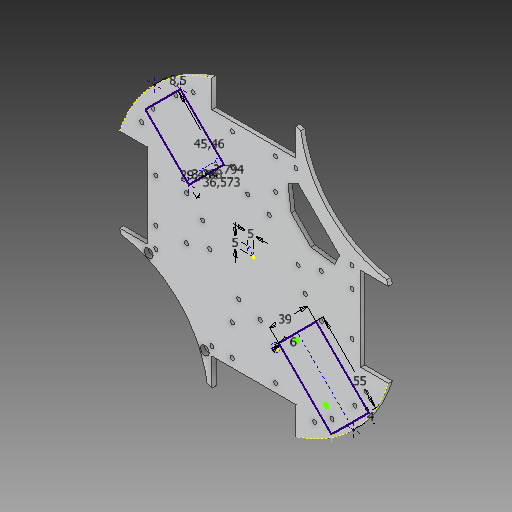
# Autodesk Inventor part: floor-01
Saved by Autodesk Inventor 2020 (Build 240168000, 168)
## iProperties
Created: 2024-09-07
Part Number: floor-01
Material: Типовые
Document SubType Name: Modeling
Designer: Ivan
Density: 1 g/cm^3
Appearance: С текстурой — серый
Author: Ivan
Autodesk Inventor part; units mm, degrees
ref_plane "YZ Plane" through (0, 0, 0) normal (1, 0, 0) x (0, 1, 0)
ref_plane "XZ Plane" through (0, 0, 0) normal (0, 1, 0) x (-1, 0, 0)
ref_plane "XY Plane" through (0, 0, 0) normal (0, 0, 1) x (1, 0, 0)
sketch "Эскиз2" plane through (0, 0, 0) normal (0, 0, 1) x (1, 0, 0)
  circle A0 centre (0, 0) radius 107.5
  circle A1 centre (0, 0) radius 104
  line L0 (-99.2724, 31) -> (-78.7724, 31)
  line L1 (-99.2724, -31) -> (-78.7724, -31)
  line L2 (-31, 99.2724) -> (-31, 78.7724)
  line L3 (31, 99.2724) -> (31, 78.7724)
  line L4 (99.2724, 31) -> (78.7724, 31)
  line L5 (99.2724, -31) -> (78.7724, -31)
  line L6 (31, -99.2724) -> (31, -78.7724)
  line L7 (-31, -99.2724) -> (-31, -78.7724)
  line L8 (-78.7724, -31) -> (-78.7724, 31)
  line L9 (-31, 78.7724) -> (31, 78.7724)
  line L10 (78.7724, 31) -> (78.7724, -31)
  line L11 (31, -78.7724) -> (-31, -78.7724)
  circle A2 centre (-109.0212, -109.0212) radius 75.25
  line L12 (-31, 78.7724) -> (78.7724, -31) construction
  line L13 (-73.5391, 73.5391) -> (73.5391, -73.5391) construction
  circle A3 centre (109.0212, 109.0212) radius 75.25
  point P0 (-98.0863, -34.57)
  point P1 (-34.57, -98.0863)
  point P2 (98.0863, 34.57)
  point P3 (34.57, 98.0863)
  dimension "d1" = 208
  dimension "d0" = 215
  dimension "d8" = 20.5
  dimension "d9" = 31
  dimension "d10" = 31
  dimension "d11" = 31
  dimension "d12" = 31
  dimension "d13" = 31
  dimension "d14" = 31
  dimension "d15" = 31
  dimension "d16" = 31
  dimension "d17" = 150.5
  dimension "d18" = 3.57
  dimension "d19" = 3.57
  constraints: 28 end point, 7 equal length, 4 horizontal, 4 vertical, 3 centre point, 2 coincident, 2 point on circle, 1 midpoint, 1 parallel, 1 symmetric about line, 15 other
  measures "d0" diameter of A0
  measures "d8" distance of L0.start L0.end
  measures "d9" distance from line of L0 point (0, 0)
  measures "d10" distance from line of L7 point (0, 0)
  measures "d11" distance from line of L6 point (0, 0)
  measures "d12" distance from line of L5 point (0, 0)
  measures "d13" distance from line of L4 point (0, 0)
  measures "d14" distance from line of L3 point (0, 0)
  measures "d15" distance from line of L2 A0.centre
  measures "d16" distance from line of L1 point (0, 0)
  measures "d17" diameter of A2
  measures "d18" vertical distance of L1.start A2.end
  measures "d19" horizontal distance of L7.start A2.start
extrude "Выдавливание1" add sketch "Эскиз2" along normal blind 3 contours A1 L4 L10 L5 L6 L11 L7 A2 L1 L8 L0 L2 L9 L3 A3
sketch "Эскиз3" plane through (0, 0, 0) normal (0, 0, -1) x (-1, 0, 0)
  line L0 (-78.7724, -31) -> (-78.7724, 31) projected
  line L1 (-78.7724, 16) -> (78.7724, 16) construction
  line L2 (78.7724, 31) -> (78.7724, -31) projected
  line L3 (-31, 78.7724) -> (31, 78.7724) projected
  line L4 (31, -78.7724) -> (-31, -78.7724) projected
  line L5 (-16, -78.7724) -> (-16, 78.7724) construction
  line L6 (0, 0) -> (0, 78.7724) construction
  line L7 (0, 0) -> (78.7724, 0) construction
  line L8 (-78.7724, -16) -> (78.7724, -16) construction
  line L9 (16, -78.7724) -> (16, 78.7724) construction
  circle A0 centre (-49.72, 16) radius 1.5
  circle A1 centre (-49.72, -16) radius 1.5
  circle A2 centre (-16, 49.72) radius 1.5
  circle A3 centre (16, 49.72) radius 1.5
  circle A4 centre (49.72, 16) radius 1.5
  circle A5 centre (49.72, -16) radius 1.5
  line L10 (-49.72, 49.72) -> (49.72, 49.72) construction
  line L11 (49.72, 49.72) -> (49.72, -49.72) construction
  line L12 (49.72, -49.72) -> (-49.72, -49.72) construction
  line L13 (-49.72, -49.72) -> (-49.72, 49.72) construction
  line L14 (-49.72, 49.72) -> (49.72, -49.72) construction
  circle A6 centre (-16, -49.72) radius 1.5
  circle A7 centre (16, -49.72) radius 1.5
  line L15 (-72.43, 72.43) -> (72.43, 72.43) construction
  line L16 (72.43, 72.43) -> (72.43, -72.43) construction
  line L17 (72.43, -72.43) -> (-72.43, -72.43) construction
  line L18 (-72.43, -72.43) -> (-72.43, 72.43) construction
  line L19 (-72.43, 72.43) -> (72.43, -72.43) construction
  circle A8 centre (-72.43, 16) radius 1.5
  circle A9 centre (-72.43, -16) radius 1.5
  circle A10 centre (-16, 72.43) radius 1.5
  circle A11 centre (16, 72.43) radius 1.5
  circle A12 centre (72.43, 16) radius 1.5
  circle A13 centre (72.43, -16) radius 1.5
  circle A14 centre (16, -72.43) radius 1.5
  circle A15 centre (-16, -72.43) radius 1.5
  circle A16 centre (-72.43, 31) radius 1.5
  circle A17 centre (-31, 72.43) radius 1.5
  circle A18 centre (31, -72.43) radius 1.5
  circle A19 centre (72.43, -31) radius 1.5
  line L20 (-99.2724, -31) -> (-78.7724, -31) projected
  line L21 (-31, -78.7724) -> (-31, -99.2724) projected
  arc A20 (-89.0224, -31) -> (-31, -89.0224) centre (0, 0) ccw construction
  arc A21 (89.0224, 31) -> (31, 89.0224) centre (0, 0) ccw construction
  circle A22 centre (-57.67, -74.5664) radius 1.5
  line L22 (-72.43, -72.43) -> (72.43, 72.43) construction
  circle A23 centre (-74.5664, -57.67) radius 1.5
  circle A24 centre (-44.87, -82.9015) radius 1.5
  circle A25 centre (-82.9015, -44.87) radius 1.5
  circle A26 centre (74.5664, 57.67) radius 1.5
  circle A27 centre (57.67, 74.5664) radius 1.5
  circle A28 centre (82.9015, 44.87) radius 1.5
  circle A29 centre (44.87, 82.9015) radius 1.5
  dimension "d22" = 16
  dimension "d23" = 16
  dimension "d25" = 99.44
  dimension "d26" = 3
  dimension "d27" = 144.86
  dimension "d28" = 3
  dimension "d29" = 3
  dimension "d30" = 15
  dimension "d31" = 15
  dimension "d32" = 15
  dimension "d33" = 15
  dimension "d35" = 26.67
  dimension "d36" = 13.87
  dimension "d37" = 3
  constraints: 39 point on line, 34 end point, 30 centre point, 18 equal radius, 12 symmetric about line, 6 midpoint, 6 point on circle, 4 parallel, 4 perpendicular, 3 horizontal, 1 coincident, 1 vertical, 7 other
  measures "d22" distance from line of L1 L6.start
  measures "d23" distance from line of L5 L6.start
  measures "d25" distance of L11.end L12.end
  measures "d26" diameter of A0
  measures "d27" distance of L17.end L15.start
  measures "d28" diameter of A11
  measures "d29" diameter of A16
  measures "d30" distance of A16.centre A8.centre
  measures "d31" distance of A17.centre A10.centre
  measures "d32" distance of A13.centre A19.centre
  measures "d33" distance of A14.centre A18.centre
  measures "d35" distance from line of L21 A22.centre
  measures "d36" distance from line of L21 A24.centre
  measures "d37" diameter of A24
extrude "Выдавливание2" cut sketch "Эскиз3" against normal blind 3
sketch "Эскиз5" plane through (0, 0, 3) normal (0, 0, 1) x (1, 0, 0)
  circle A0 centre (16, -72.43) radius 1.5 projected
  circle A1 centre (16, -49.72) radius 1.5 projected
  circle A2 centre (49.72, -16) radius 1.5 projected
  circle A3 centre (49.72, 16) radius 1.5 projected
  circle A4 centre (72.43, 31) radius 1.5 projected
  circle A5 centre (-44.87, 82.9015) radius 1.5 projected
  circle A6 centre (57.67, -74.5664) radius 1.5 projected
  circle A7 centre (31, 72.43) radius 1.5 projected
  circle A8 centre (-57.67, 74.5664) radius 1.5 projected
  circle A9 centre (72.43, 16) radius 1.5 projected
  circle A10 centre (-49.72, 16) radius 1.5 projected
  circle A11 centre (-49.72, -16) radius 1.5 projected
  circle A12 centre (-16, -49.72) radius 1.5 projected
  circle A13 centre (74.5664, -57.67) radius 1.5 projected
  circle A14 centre (-16, -72.43) radius 1.5 projected
  circle A15 centre (-72.43, -31) radius 1.5 projected
  circle A16 centre (72.43, -16) radius 1.5 projected
  circle A17 centre (16, 49.72) radius 1.5 projected
  circle A18 centre (-82.9015, 44.87) radius 1.5 projected
  circle A19 centre (-16, 72.43) radius 1.5 projected
  circle A20 centre (44.87, -82.9015) radius 1.5 projected
  circle A21 centre (16, 72.43) radius 1.5 projected
  circle A22 centre (-74.5664, 57.67) radius 1.5 projected
  circle A23 centre (-16, 49.72) radius 1.5 projected
  circle A24 centre (-72.43, 16) radius 1.5 projected
  circle A25 centre (-72.43, -16) radius 1.5 projected
  circle A26 centre (-31, -72.43) radius 1.5 projected
  circle A27 centre (82.9015, -44.87) radius 1.5 projected
  arc A28 (-34.57, -98.0863) -> (-98.0863, -34.57) centre (-109.0212, -109.0212) ccw projected
  arc A29 (-34.57, -98.0863) -> (-31, -99.2724) centre (0, 0) ccw projected
  line L0 (-31, -99.2724) -> (-31, -78.7724) projected
  line L1 (-31, -78.7724) -> (31, -78.7724) projected
  line L2 (31, -78.7724) -> (31, -99.2724) projected
  arc A30 (31, -99.2724) -> (99.2724, -31) centre (0, 0) ccw projected
  line L3 (99.2724, -31) -> (78.7724, -31) projected
  line L4 (78.7724, -31) -> (78.7724, 31) projected
  line L5 (78.7724, 31) -> (99.2724, 31) projected
  arc A31 (99.2724, 31) -> (98.0863, 34.57) centre (0, 0) ccw projected
  arc A32 (34.57, 98.0863) -> (98.0863, 34.57) centre (109.0212, 109.0212) ccw projected
  arc A33 (34.57, 98.0863) -> (31, 99.2724) centre (0, 0) ccw projected
  line L6 (31, 99.2724) -> (31, 78.7724) projected
  line L7 (31, 78.7724) -> (-31, 78.7724) projected
  line L8 (-31, 78.7724) -> (-31, 99.2724) projected
  arc A34 (-31, 99.2724) -> (-99.2724, 31) centre (0, 0) ccw projected
  line L9 (-99.2724, 31) -> (-78.7724, 31) projected
  line L10 (-78.7724, 31) -> (-78.7724, -31) projected
  line L11 (-78.7724, -31) -> (-99.2724, -31) projected
  arc A35 (-99.2724, -31) -> (-98.0863, -34.57) centre (0, 0) ccw projected
  arc A36 (-31, 99.2724) -> (-99.2724, 31) centre (0, 0) ccw projected
  arc A37 (-31, 99.2724) -> (-99.2724, 31) centre (0, 0) ccw
  arc A38 (31, -99.2724) -> (99.2724, -31) centre (0, 0) ccw projected
  arc A39 (31, -99.2724) -> (99.2724, -31) centre (0, 0) ccw
  arc A40 (-34.57, -98.0863) -> (-98.0863, -34.57) centre (-109.0212, -109.0212) ccw projected
  arc A41 (-34.57, -98.0863) -> (-98.0863, -34.57) centre (-109.0212, -109.0212) ccw
  arc A42 (34.57, 98.0863) -> (98.0863, 34.57) centre (109.0212, 109.0212) ccw projected
  arc A43 (34.57, 98.0863) -> (98.0863, 34.57) centre (109.0212, 109.0212) ccw
  arc A44 (34.57, 98.0863) -> (31, 99.2724) centre (0, 0) ccw projected
  arc A45 (34.57, 98.0863) -> (31, 99.2724) centre (0, 0) ccw
  arc A46 (99.2724, 31) -> (98.0863, 34.57) centre (0, 0) ccw projected
  arc A47 (99.2724, 31) -> (98.0863, 34.57) centre (0, 0) ccw
  arc A48 (-34.57, -98.0863) -> (-31, -99.2724) centre (0, 0) ccw projected
  arc A49 (-34.57, -98.0863) -> (-31, -99.2724) centre (0, 0) ccw
  arc A50 (-99.2724, -31) -> (-98.0863, -34.57) centre (0, 0) ccw projected
  arc A51 (-99.2724, -31) -> (-98.0863, -34.57) centre (0, 0) ccw
  line L12 (-99.2724, 31) -> (-78.7724, 31) projected
  line L13 (-99.2724, 31) -> (-78.7724, 31)
  line L14 (-78.7724, 31) -> (-78.7724, -31) projected
  line L15 (-78.7724, 31) -> (-78.7724, -31)
  line L16 (-78.7724, -31) -> (-99.2724, -31)
  line L17 (-78.7724, -31) -> (-99.2724, -31) projected
  line L18 (-78.7724, -31) -> (-99.2724, -31)
  line L19 (-31, 78.7724) -> (-31, 99.2724) projected
  line L20 (-31, 99.2724) -> (-31, 78.7724)
  line L21 (31, 78.7724) -> (-31, 78.7724) projected
  line L22 (-31, 78.7724) -> (31, 78.7724)
  line L23 (31, 99.2724) -> (31, 78.7724) projected
  line L24 (31, 78.7724) -> (31, 99.2724)
  line L25 (78.7724, 31) -> (99.2724, 31) projected
  line L26 (99.2724, 31) -> (78.7724, 31)
  line L27 (78.7724, -31) -> (78.7724, 31) projected
  line L28 (78.7724, 31) -> (78.7724, -31)
  line L29 (99.2724, -31) -> (78.7724, -31) projected
  line L30 (78.7724, -31) -> (99.2724, -31)
  line L31 (-31, -99.2724) -> (-31, -78.7724) projected
  line L32 (-31, -99.2724) -> (-31, -78.7724)
  line L33 (-31, -78.7724) -> (31, -78.7724) projected
  line L34 (-31, -78.7724) -> (31, -78.7724)
  line L35 (31, -78.7724) -> (31, -99.2724)
  circle A52 centre (-49.72, 16) radius 1.5
  circle A53 centre (-72.43, 16) radius 1.5
  circle A54 centre (-49.72, -16) radius 1.5
  circle A55 centre (-72.43, -16) radius 1.5
  circle A56 centre (-72.43, -31) radius 1.5
  circle A57 centre (-16, -49.72) radius 1.5 projected
  circle A58 centre (-16, -49.72) radius 1.5
  circle A59 centre (-31, -72.43) radius 1.5 projected
  circle A60 centre (-31, -72.43) radius 1.5
  circle A61 centre (-16, -72.43) radius 1.5
  circle A62 centre (16, -72.43) radius 1.5 projected
  circle A63 centre (16, -72.43) radius 1.5
  circle A64 centre (44.87, -82.9015) radius 1.5
  circle A65 centre (57.67, -74.5664) radius 1.5
  circle A66 centre (16, -49.72) radius 1.5
  circle A67 centre (74.5664, -57.67) radius 1.5
  circle A68 centre (82.9015, -44.87) radius 1.5
  circle A69 centre (49.72, -16) radius 1.5
  circle A70 centre (72.43, -16) radius 1.5
  circle A71 centre (72.43, 16) radius 1.5
  circle A72 centre (49.72, 16) radius 1.5
  circle A73 centre (72.43, 31) radius 1.5
  circle A74 centre (31, 72.43) radius 1.5
  circle A75 centre (16, 72.43) radius 1.5
  circle A76 centre (16, 49.72) radius 1.5
  circle A77 centre (-16, 49.72) radius 1.5
  circle A78 centre (-16, 72.43) radius 1.5
  circle A79 centre (-44.87, 82.9015) radius 1.5
  circle A80 centre (-57.67, 74.5664) radius 1.5
  circle A81 centre (-74.5664, 57.67) radius 1.5
  circle A82 centre (-82.9015, 44.87) radius 1.5
  constraints: 36 centre point, 36 coincident, 26 end point, 19 concentric, 17 point on circle, 9 collinear, 1 horizontal, 1 perpendicular, 1 point on line
hole "Отверстие1" at (0, 0, 3) direction (0, 0, -1) diameter 40 end through all
sketch "Эскиз8" plane through (0, 0, 3) normal (0, 0, 1) x (1, 0, 0)
  circle A0 centre (-48.1257, 27.2915) radius 1.397 construction
  circle A1 centre (-27.2915, 48.1257) radius 1.397 construction
  line L0 (-48.3138, 22.4528) -> (-22.4528, 48.3138)
  line L1 (-22.4528, 48.3138) -> (-54.5982, 80.4592)
  line L2 (-54.5982, 80.4592) -> (-80.4592, 54.5982)
  line L3 (-80.4592, 54.5982) -> (-48.3138, 22.4528)
  line L4 (-27.2915, 48.1257) -> (-48.1257, 27.2915) construction
  line L5 (-37.7086, 37.7086) -> (-35.3833, 35.3833) construction
  arc A2 (-31, 99.2724) -> (-99.2724, 31) centre (0, 0) ccw construction
  line L6 (0, 0) -> (-5, 0) construction
  line L7 (-5, 0) -> (-5, 5) construction
  line L8 (-5, 5) -> (0, 5) construction
  line L9 (0, 5) -> (0, 0) construction
  line L10 (0, 0) -> (-5, 5) construction
  line L11 (84.4993, -56.9221) -> (56.9221, -84.4993)
  line L12 (56.9221, -84.4993) -> (18.0312, -45.6084)
  line L13 (18.0312, -45.6084) -> (45.6084, -18.0312)
  line L14 (45.6084, -18.0312) -> (84.4993, -56.9221)
  line L15 (31.8198, -31.8198) -> (70.7107, -70.7107) construction
  arc A3 (31, -99.2724) -> (99.2724, -31) centre (0, 0) ccw construction
  circle A4 centre (53.033, -67.8823) radius 1.6
  circle A5 centre (31.2924, -37.2462) radius 1.6
  circle A6 centre (16, -49.72) radius 1.5 projected
  circle A7 centre (16, -49.72) radius 1.5 projected
  circle A8 centre (16, -49.72) radius 3 construction
  point P0 (-73.5391, 73.5391)
  point P1 (73.5391, -73.5391)
  dimension "d47" = 45.4604
  dimension "d48" = 36.573
  dimension "d49" = 2.794
  dimension "d50" = 29.464
  dimension "d52" = 5
  dimension "d53" = 5
  dimension "d54" = 3.2884
  dimension "d55" = 8.5
  dimension "d58" = 39
  dimension "d62" = 4
  dimension "d79" = 55
  dimension "d80" = 6
  constraints: 32 end point, 6 parallel, 5 centre point, 5 perpendicular, 4 midpoint, 2 collinear, 2 point on circle, 1 coincident, 1 equal radius, 1 horizontal
  measures "d47" distance of L0.end L1.end
  measures "d48" distance of L0.start L0.end
  measures "d49" diameter of A1
  measures "d50" distance of L4.start L4.end
  measures "d52" distance of L7.end L8.end
  measures "d53" distance of L6.end L7.end
  measures "d54" distance from line of L0 L5.start
  measures "d55" distance from line of L2 point (-73.539, 73.539)
  measures "d58" distance of L12.end L13.end
  measures "d62" distance from line of L11 point (73.539, -73.539)
  measures "d79" distance from line of L11 L13.end
  measures "d80" diameter of A8
sketch "Эскиз10" plane through (0, 0, 3) normal (0, 0, 1) x (1, 0, 0)
  point P0 (0, 0)
sketch "Эскиз11" plane through (0, 0, 3) normal (0, 0, 1) x (1, 0, 0)
  circle A0 centre (0, 0) radius 20 projected
  circle A1 centre (16, -72.43) radius 1.5 projected
  circle A2 centre (16, -49.72) radius 1.5 projected
  circle A3 centre (49.72, -16) radius 1.5 projected
  circle A4 centre (49.72, 16) radius 1.5 projected
  circle A5 centre (72.43, 31) radius 1.5 projected
  circle A6 centre (-44.87, 82.9015) radius 1.5 projected
  circle A7 centre (31, 72.43) radius 1.5 projected
  circle A8 centre (72.43, 16) radius 1.5 projected
  circle A9 centre (-49.72, 16) radius 1.5 projected
  circle A10 centre (-49.72, -16) radius 1.5 projected
  circle A11 centre (-16, -49.72) radius 1.5 projected
  circle A12 centre (-16, -72.43) radius 1.5 projected
  circle A13 centre (-72.43, -31) radius 1.5 projected
  circle A14 centre (72.43, -16) radius 1.5 projected
  circle A15 centre (16, 49.72) radius 1.5 projected
  circle A16 centre (-82.9015, 44.87) radius 1.5 projected
  circle A17 centre (-16, 72.43) radius 1.5 projected
  circle A18 centre (44.87, -82.9015) radius 1.5 projected
  circle A19 centre (16, 72.43) radius 1.5 projected
  circle A20 centre (-16, 49.72) radius 1.5 projected
  circle A21 centre (-72.43, 16) radius 1.5 projected
  circle A22 centre (-72.43, -16) radius 1.5 projected
  circle A23 centre (-31, -72.43) radius 1.5 projected
  circle A24 centre (82.9015, -44.87) radius 1.5 projected
  arc A25 (-34.57, -98.0863) -> (-98.0863, -34.57) centre (-109.0212, -109.0212) ccw projected
  arc A26 (-34.57, -98.0863) -> (-31, -99.2724) centre (0, 0) ccw projected
  line L0 (-31, -99.2724) -> (-31, -78.7724) projected
  line L1 (-31, -78.7724) -> (31, -78.7724) projected
  line L2 (31, -78.7724) -> (31, -99.2724) projected
  arc A27 (31, -99.2724) -> (99.2724, -31) centre (0, 0) ccw projected
  line L3 (99.2724, -31) -> (78.7724, -31) projected
  line L4 (78.7724, -31) -> (78.7724, 31) projected
  line L5 (78.7724, 31) -> (99.2724, 31) projected
  arc A28 (99.2724, 31) -> (98.0863, 34.57) centre (0, 0) ccw projected
  arc A29 (34.57, 98.0863) -> (98.0863, 34.57) centre (109.0212, 109.0212) ccw projected
  arc A30 (34.57, 98.0863) -> (31, 99.2724) centre (0, 0) ccw projected
  line L6 (31, 99.2724) -> (31, 78.7724) projected
  line L7 (31, 78.7724) -> (-31, 78.7724) projected
  line L8 (-31, 78.7724) -> (-31, 99.2724) projected
  arc A31 (-31, 99.2724) -> (-99.2724, 31) centre (0, 0) ccw projected
  line L9 (-99.2724, 31) -> (-78.7724, 31) projected
  line L10 (-78.7724, 31) -> (-78.7724, -31) projected
  line L11 (-78.7724, -31) -> (-99.2724, -31) projected
  arc A32 (-99.2724, -31) -> (-98.0863, -34.57) centre (0, 0) ccw projected
  circle A33 centre (-27.2915, 48.1257) radius 1.397 construction
  circle A34 centre (-48.1257, 27.2915) radius 1.397 construction
  circle A35 centre (-27.2915, 48.1257) radius 1.397
  circle A36 centre (-48.1257, 27.2915) radius 1.397
  circle A37 centre (31.2924, -37.2462) radius 1.6 projected
  circle A38 centre (53.033, -67.8823) radius 1.6 projected
  constraints: 2 centre point, 2 coincident, 2 concentric
sketch "Эскиз12" plane through (0, 0, 3) normal (0, 0, 1) x (1, 0, 0)
  circle A0 centre (-72.43, -31) radius 3.3 construction
  circle A1 centre (-72.43, -16) radius 3.3 construction
  circle A2 centre (-31, -72.43) radius 3.3 construction
  circle A3 centre (-16, -72.43) radius 3.3 construction
  line L0 (-72.43, -31) -> (-72.43, -16) construction
  line L1 (-31, -72.43) -> (-16, -72.43) construction
  line L2 (-32.6924, -63.2376) -> (-63.2376, -32.6924)
  circle A4 centre (-16, -42.22) radius 3.3 construction
  circle A5 centre (-42.22, -16) radius 3.3 construction
  line L3 (-16, -42.22) -> (-42.22, -16) construction
  line L4 (-42.0023, -27.4404) -> (-59.5377, -25.1696)
  line L5 (-27.4404, -42.0023) -> (-25.1696, -59.5377)
  line L6 (-63.2376, -32.6924) -> (-59.5377, -25.1696) construction
  line L7 (-32.6924, -63.2376) -> (-25.1696, -59.5377) construction
  line L8 (-27.4404, -42.0023) -> (-42.0023, -27.4404) construction
  line L9 (-27.4404, -42.0023) -> (-42.0023, -27.4404)
  line L10 (-59.5377, -25.1696) -> (-63.2376, -32.6924)
  line L11 (-32.6924, -63.2376) -> (-25.1696, -59.5377)
  line L12 (32.6924, 63.2376) -> (63.2376, 32.6924)
  line L13 (42.0023, 27.4404) -> (59.5377, 25.1696)
  line L14 (63.2376, 32.6924) -> (59.5377, 25.1696)
  line L15 (32.6924, 63.2376) -> (25.1696, 59.5377)
  line L16 (27.4404, 42.0023) -> (25.1696, 59.5377)
  line L17 (27.4404, 42.0023) -> (42.0023, 27.4404)
  point P0 (0, 0)
  point P1 (0, 0)
  point P2 (-23.5, -72.43)
  point P3 (-72.43, -23.5)
  point P4 (-29.11, -29.11)
  point P5 (72.43, 23.5)
  point P6 (23.5, 72.43)
  point P7 (29.11, 29.11)
  dimension "d65" = 13
  dimension "d66" = 13
  dimension "d67" = 13
  dimension "d68" = 13
  dimension "d69" = 13
  dimension "d70" = 13
  dimension "d71" = 360
  constraints: 36 end point, 12 point on line, 6 centre point, 3 midpoint, 2 collinear, 1 horizontal, 1 vertical, 31 other
  measures "d65" distance of L2.end point (-72.43, -23.5)
  measures "d66" distance of L4.end point (-72.43, -23.5)
  measures "d67" distance of L2.start point (-23.5, -72.43)
  measures "d68" distance of L5.end point (-23.5, -72.43)
  measures "d69" distance of L5.start point (-29.11, -29.11)
  measures "d70" distance of L4.start point (-29.11, -29.11)
extrude "Выдавливание4" cut sketch "Эскиз12" against normal blind 10 contours L12 L14 L13 L17 L16 L15
extrude "Выдавливание5" add sketch "Эскиз11" against normal up to surface (3 mm away) contours A0
sketch "Эскиз14" plane through (0, 0, 0) normal (0, 0, -1) x (-1, 0, 0)
  line L0 (-11.9501, 37.5474) -> (-37.5474, 11.9501)
  line L1 (-37.5474, 11.9501) -> (11.9501, -37.5474)
  line L2 (11.9501, -37.5474) -> (37.5474, -11.9501)
  line L3 (37.5474, -11.9501) -> (-11.9501, 37.5474)
  line L4 (-11.9501, 37.5474) -> (11.9501, -37.5474) construction
  line L5 (-11.243, 32.5976) -> (32.5976, -11.243)
  line L6 (0, 0) -> (6.2542, 6.2542) construction
  circle A0 centre (-11.243, 32.5976) radius 1.5
  line L7 (0, 0) -> (-6.2542, 6.2542) construction
  line L8 (0, 0) -> (9.1217, 2.0506) construction
  circle A1 centre (-32.5976, 11.243) radius 1.5
  circle A2 centre (32.5976, -11.243) radius 1.5
  circle A3 centre (11.243, -32.5976) radius 1.5
  line L9 (-31, 78.7724) -> (31, 78.7724) construction
  line L10 (99.2724, 31) -> (78.7724, 31) construction
  line L11 (31, 78.7724) -> (78.7724, 31) construction
  point P0 (10.6773, 10.6773)
  point P1 (9.1217, 9.1217)
  dimension "d81" = 36.2
  dimension "d82" = 70
  dimension "d83" = 4
  dimension "d84" = 3
  dimension "d85" = 3
  constraints: 20 end point, 4 centre point, 4 parallel, 3 coincident, 3 symmetric about line, 2 midpoint, 2 perpendicular, 2 point on line, 3 other
  measures "d81" distance of L2.end L1.end
  measures "d82" distance of L1.end L0.end
  measures "d83" distance from line of L0 L5.start
  measures "d84" distance from line of L3 point (10.677, 10.677)
  measures "d85" diameter of A0
hole "Отверстие2" at (11.243, 32.5976, 0) at (32.5976, 11.243, 0) at (-32.5976, -11.243, 0) at (-11.243, -32.5976, 0) direction (0, 0, 1) diameter 3 end through all
sketch "Эскиз15" plane through (0, 0, 3) normal (0, 0, 1) x (1, 0, 0)
  circle A0 centre (124.1994, 64.0459) radius 3
  circle A1 centre (-31, -72.43) radius 1.5
  circle A2 centre (-72.43, -31) radius 1.5
  line L0 (-72.43, -31) -> (-31, -72.43)
  line L1 (-31, -72.43) -> (-36.2927, -77.7227)
  circle A3 centre (-36.2927, -77.7227) radius 2
  line L2 (164.6688, 164.6688) -> (-154.6363, -154.6363)
  circle A4 centre (-77.7227, -36.2927) radius 2
  point P0 (0, 0)
  point P1 (0, 0)
  point P2 (129.0863, 44.2024)
  dimension "d94" = 6
  dimension "d95" = 7.485
  dimension "d96" = 4
  constraints: 6 end point, 5 centre point, 1 coincident, 1 perpendicular, 1 symmetric about line, 1 other
  measures "d94" diameter of A0
  measures "d95" distance from line of L0 L1.end
  measures "d96" diameter of A3
hole "Отверстие3" at (-77.7227, -36.2927, 3) at (-36.2927, -77.7227, 3) direction (0, 0, -1) diameter 6.5 end through all
sketch "Эскиз16" plane through (0, 0, 3) normal (0, 0, 1) x (1, 0, 0)
  circle A0 centre (49.1515, 117.5129) radius 1.65
  circle A1 centre (49.1515, 117.5129) radius 3.35
  circle A2 centre (3.9014, 156.8484) radius 1.65
  circle A3 centre (80, 152.9999) radius 1.65
  circle A4 centre (34.7499, 192.3354) radius 1.65
  circle A5 centre (41.9507, 154.9241) radius 41.494
  line L0 (45.9767, 118.5821) -> (51.7025, 119.6842)
  arc A6 (39.3031, 113.5146) -> (45.9767, 118.5821) centre (26.7374, 136.9912) ccw
  arc A7 (51.7025, 119.6842) -> (59.7803, 117.456) centre (62.7338, 143.9197) ccw
  arc A8 (78.4993, 155.995) -> (82.5887, 163.3089) centre (57.5919, 172.4852) ccw
  circle A9 centre (80, 152.9999) radius 3.35
  arc A10 (81.5355, 142.4824) -> (78.2048, 150.1715) centre (55.7405, 135.8747) ccw
  arc A11 (5.402, 153.8533) -> (1.3126, 146.5394) centre (26.3095, 137.3631) ccw
  circle A12 centre (3.9014, 156.8484) radius 3.35
  arc A13 (2.3659, 167.3659) -> (5.6965, 159.6768) centre (28.1609, 173.9736) ccw
  arc A14 (32.1989, 190.1641) -> (24.1211, 192.3923) centre (21.1675, 165.9286) ccw
  circle A15 centre (34.7499, 192.3354) radius 3.35
  arc A16 (44.5983, 196.3336) -> (37.9247, 191.2662) centre (57.1641, 172.8571) ccw
  line L1 (39.3031, 113.5146) -> (59.7803, 117.456) construction
  line L2 (-47.0226, -10.253) -> (10.253, 47.0226) construction
  line L3 (2.3659, 167.3659) -> (59.7803, 117.456) construction
  line L4 (24.121, 192.3922) -> (81.5355, 142.4824) construction
  line L5 (1.3126, 146.5394) -> (44.5983, 196.3336) construction
  line L6 (82.5887, 163.3089) -> (39.3031, 113.5146) construction
  circle A17 centre (41.9507, 154.9241) radius 38.0979 construction
  line L7 (45.9767, 118.5821) -> (46.9111, 113.7277) construction
  line L8 (78.2048, 150.1715) -> (78.4993, 155.995) construction
  line L9 (41.9507, 154.9241) -> (80, 152.9999) construction
  line L10 (41.9507, 154.9241) -> (34.7499, 192.3354) construction
  line L11 (41.9507, 154.9241) -> (3.9014, 156.8484) construction
  line L12 (5.6965, 159.6768) -> (5.402, 153.8533) construction
  line L13 (32.1989, 190.1641) -> (37.9247, 191.2662) construction
  line L14 (41.9507, 154.9241) -> (49.1515, 117.5129) construction
  circle A18 centre (-37.8224, 4.5736) radius 3.3
  circle A19 centre (-4.5736, 37.8224) radius 3.3
  circle A20 centre (4.5736, -37.8224) radius 3.3
  circle A21 centre (37.8224, -4.5736) radius 3.3
  circle A22 centre (16, -49.72) radius 3.3
  line L15 (-37.8224, 4.5736) -> (-4.5736, 37.8224) construction
  line L16 (4.5736, -37.8224) -> (37.8224, -4.5736) construction
  line L17 (-21.198, 21.198) -> (21.198, -21.198) construction
  line L18 (-4.5736, 37.8224) -> (37.8224, -4.5736) construction
  point P0 (0, 0)
  point P1 (0, 0)
  point P2 (-47.6168, 71.9305)
  point P3 (-60.3824, 55.6528)
  point P4 (-60.3824, 22.3934)
  point P5 (-47.6168, 6.1158)
  point P6 (2.7831, 6.1158)
  point P7 (15.5487, 22.3934)
  point P8 (15.2441, 55.8587)
  point P9 (2.9104, 71.5855)
  point P10 (0, 0)
  dimension "d106" = 82.9881
  dimension "d104" = 3.3
  dimension "d105" = 6.7
  dimension "d107" = 26.6279
  dimension "d108" = 20.4772
  dimension "d109" = 3.7148
  dimension "d110" = 33.1603
  dimension "d111" = 50.338
  dimension "d112" = 16.5802
  dimension "d113" = 25.169
  dimension "d114" = 10.4265
  dimension "d115" = 10.4265
  dimension "d116" = 10.4265
  dimension "d117" = 10.4265
  dimension "d118" = 10.4265
  dimension "d119" = 10.4265
  dimension "d120" = 59.957
  dimension "d121" = 47.021
  constraints: 38 end point, 28 point on circle, 22 centre point, 13 equal radius, 9 perpendicular, 6 coincident, 4 equal length, 4 parallel, 3 midpoint, 1 tangent, 12 other
  measures "d104" diameter of A0
  measures "d105" diameter of A1
  measures "d107" radius of A6
  measures "d108" horizontal distance of L1.end L1.start
  measures "d109" distance from line of L1 L0.start
  measures "d110" distance from line of L4 L3.start
  measures "d111" distance from line of L5 L6.start
  measures "d112" distance from line of L3 point (41.951, 154.924)
  measures "d113" distance from line of L5 point (41.951, 154.924)
  measures "d114" distance from line of L9 L6.start
  measures "d115" distance from line of L9 A10.start
  measures "d116" distance from line of L10 A14.end
  measures "d117" distance from line of L10 L5.end
  measures "d118" distance from line of L11 L3.start
  measures "d119" distance from line of L14 L1.end
  measures "d120" distance from line of L15 L16.end
  measures "d121" distance from line of L18 L15.start
hole "Отверстие4" at (-4.5736, 37.8224, 3) at (37.8224, -4.5736, 3) at (4.5736, -37.8224, 3) at (-37.8224, 4.5736, 3) direction (0, 0, -1) diameter 3 end through all
